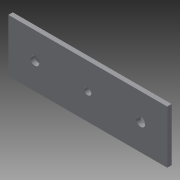
# Autodesk Inventor part: PistonPlate_v1
Saved by Autodesk Inventor 2013 (Build 170138000, 138)
## iProperties
Created: 2013-01-23
Part Number: PistonPlate_v1
Material: Generic
Document SubType Name: Modeling
Designer: motoennies
Density: 1 g/cm^3
Author: motoennies
Autodesk Inventor part; units mm, degrees
ref_plane "YZ Plane" through (0, 0, 0) normal (1, 0, 0) x (0, 1, 0)
ref_plane "XZ Plane" through (0, 0, 0) normal (0, 1, 0) x (-1, 0, 0)
ref_plane "XY Plane" through (0, 0, 0) normal (0, 0, 1) x (1, 0, 0)
sketch "Sketch1" plane through (0, 0, 0) normal (0, 0, 1) x (1, 0, 0)
  line L0 (0, 0) -> (0, 38.1)
  line L1 (0, 38.1) -> (114.3, 38.1)
  line L2 (114.3, 38.1) -> (114.3, 0)
  line L3 (0, 0) -> (114.3, 0)
  dimension "d0" = 38.1
  dimension "d1" = 114.3
  constraints: 8 end point, 2 perpendicular, 1 parallel, 1 vertical
  measures "d0" distance of L0.start L0.end
  measures "d1" distance of L0.end L1.end
extrude "Extrusion1" add sketch "Sketch1" along normal blind 3.175
sketch "Sketch2" plane through (0, 0, 3.175) normal (0, 0, 1) x (1, 0, 0)
  line L0 (114.3, 0) -> (114.3, 38.1) projected
  line L1 (114.3, 38.1) -> (0, 38.1) projected
  circle A0 centre (57.15, 19.05) radius 2.54
  line L2 (0, 38.1) -> (0, 0) projected
  circle A1 centre (19.05, 19.05) radius 3.175
  circle A2 centre (95.25, 19.05) radius 3.175
  dimension "d4" = 5.08
  dimension "d5" = 19.05
  dimension "d6" = 57.15
  dimension "d9" = 6.35
  dimension "d10" = 6.35
  dimension "d11" = 19.05
  dimension "d12" = 19.05
  constraints: 3 centre point
  measures "d4" diameter of A0
  measures "d5" distance from line of L1 A0.centre
  measures "d6" distance from line of L0 A0.centre
  measures "d9" diameter of A1
  measures "d10" diameter of A2
  measures "d11" distance from line of L2 A1.centre
  measures "d12" distance from line of L0 A2.centre
extrude "Extrusion3" cut sketch "Sketch2" against normal blind 25.4
body "Solid1"
